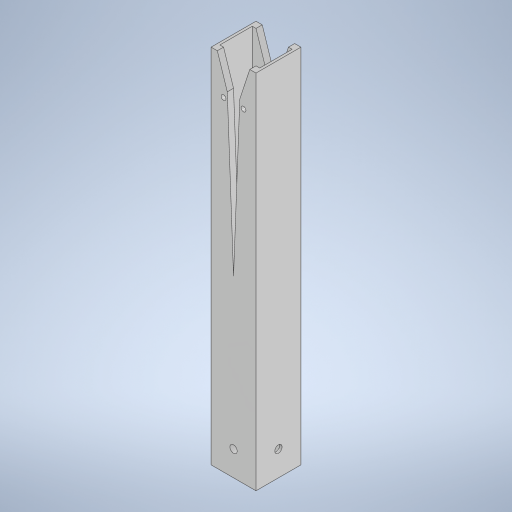
# Autodesk Inventor part: square_bar
Saved by Autodesk Inventor 2024 (Build 280153000, 153)
## iProperties
Created: 2025-01-22
Part Number: square_bar
Material: アルミニウム 6061
Document SubType Name: Modeling
Designer: 1412z
Density: 2.7 g/cm^3
Appearance: アルミニウム - つや出し
Author: 1412z
Autodesk Inventor part; units mm, degrees
ref_plane "YZ Plane" through (0, 0, 0) normal (1, 0, 0) x (0, 1, 0)
ref_plane "XZ Plane" through (0, 0, 0) normal (0, 1, 0) x (-1, 0, 0)
ref_plane "XY Plane" through (0, 0, 0) normal (0, 0, 1) x (1, 0, 0)
sketch "スケッチ1" plane through (0, 0, 0) normal (0, 1, 0) x (-1, 0, 0)
  line L0 (9, 9) -> (-9, 9)
  line L1 (-9, 9) -> (-9, -9)
  line L2 (-9, -9) -> (9, -9)
  line L3 (9, -9) -> (9, 9)
  line L4 (9, 9) -> (-9, -9) construction
  line L5 (-9, 9) -> (9, -9) construction
  point P0 (0, 0)
  dimension "d0" = 18
  dimension "d1" = 18
  constraints: 12 end point, 2 midpoint, 2 parallel, 1 horizontal, 1 perpendicular
  measures "d0" distance of L2.end L1.end
  measures "d1" distance of L1.end L0.end
extrude "押し出し1" add sketch "スケッチ1" against normal blind 150
sketch "スケッチ2" plane through (0, 0, 0) normal (0, 1, 0) x (1, 0, 0)
  line L0 (-8, -6.5) -> (8, -6.5)
  line L1 (8, -6.5) -> (8, 6.5)
  line L2 (8, 6.5) -> (-8, 6.5)
  line L3 (-8, 6.5) -> (-8, -6.5)
  line L4 (-8, -6.5) -> (8, 6.5) construction
  line L5 (8, -6.5) -> (-8, 6.5) construction
  point P0 (0, 0)
  dimension "d4" = 16
  dimension "d5" = 13
  constraints: 12 end point, 2 midpoint, 2 parallel, 1 horizontal, 1 perpendicular
  measures "d4" distance of L2.end L1.end
  measures "d5" distance of L1.end L0.end
extrude "押し出し2" cut sketch "スケッチ2" against normal blind 150
sketch "スケッチ4" plane through (-9, -150, 9) normal (0, 0, 1) x (1, 0, 0)
  circle A0 centre (5, 135) radius 1
  circle A1 centre (13, 135) radius 1
  point P0 (9, 150)
  dimension "d11" = 2
  dimension "d12" = 2
  constraints: 2 centre point
  measures "d11" diameter of A0
  measures "d12" diameter of A1
extrude "押し出し4" cut sketch "スケッチ4" against normal blind 150
sketch "スケッチ5" plane through (-9, -150, 9) normal (0, 0, 1) x (1, 0, 0)
  circle A0 centre (9, 15) radius 1.5
  point P0 (9, 150)
  dimension "d15" = 3
  constraints: 1 centre point
  measures "d15" diameter of A0
extrude "押し出し5" cut sketch "スケッチ5" against normal blind 150
sketch "スケッチ6" plane through (-9, 0, -9) normal (-1, 0, 0) x (0, 0, 1)
  circle A0 centre (9, -135) radius 1.5
  point P0 (9, 0)
  dimension "d18" = 3
  constraints: 1 centre point
  measures "d18" diameter of A0
extrude "押し出し6" cut sketch "スケッチ6" against normal blind 150
thread "ねじ1" size "M3x0.5" class "6H" standard "ANSI Metric M Profile" full length
thread "ねじ2" size "M3x0.5" class "6H" standard "ANSI Metric M Profile" full length
sketch "スケッチ7" plane through (-9, 0, 9) normal (0, 0, 1) x (1, 0, 0)
  line L0 (9, 0) -> (9, -75)
  line L1 (9, 0) -> (6, 0)
  line L2 (0, 0) -> (18, 0) projected
  line L3 (6, 0) -> (9, -75)
  line L4 (9, 0) -> (12, 0)
  line L5 (12, 0) -> (9, -75)
  point P0 (12, 0)
  dimension "d25" = 75
  dimension "d26" = 3
  dimension "d27" = 3
  constraints: 10 end point, 2 point on line, 1 vertical
  measures "d25" distance of L0.start L0.end
  measures "d26" distance of L0.start L1.end
  measures "d27" distance of L0.start L4.end
extrude "押し出し7" cut sketch "スケッチ7" against normal blind 30
sketch "スケッチ8" plane through (-9, -150, 9) normal (0, 0, 1) x (1, 0, 0)
  line L0 (9, 150) -> (15.5, 150)
  line L1 (18, 150) -> (12, 150) projected
  line L2 (9, 150) -> (9, 130)
  line L3 (9, 130) -> (15.5, 150)
  line L4 (9, 150) -> (2.5, 150)
  line L5 (2.5, 150) -> (9, 130)
  dimension "d30" = 6.5
  dimension "d31" = 20
  dimension "d32" = 6.5
  constraints: 10 end point, 1 perpendicular, 1 point on line, 1 vertical
  measures "d30" distance of L0.start L0.end
  measures "d31" distance of L0.start L2.end
  measures "d32" distance of L0.start L4.end
extrude "押し出し8" cut sketch "スケッチ8" against normal blind 30
sketch "スケッチ9" plane through (9, -150, -9) normal (0, 0, -1) x (-1, 0, 0)
  line L0 (9, 150) -> (9, 20)
  line L1 (11.5088, 137.7193) -> (9, 75) projected
  line L2 (11.5088, 137.7193) -> (11.5088, 20)
  line L3 (11.5088, 20) -> (9, 20)
  line L4 (2.5, 150) -> (6.4912, 137.7193) projected
  line L5 (6.4912, 137.7193) -> (6.4912, 20)
  line L6 (6.4912, 20) -> (9, 20)
  line L7 (6.4912, 137.7193) -> (11.5088, 137.7193)
  dimension "d35" = 130
  constraints: 12 end point, 3 perpendicular, 2 vertical, 1 parallel, 1 point on line
  measures "d35" distance of L0.start L0.end
extrude "押し出し9" cut sketch "スケッチ9" against normal blind 10
sketch "スケッチ10" plane through (0, -150, 0) normal (0, -1, 0) x (1, 0, 0)
  line L0 (-9, -9) -> (-9, 9) projected
  line L1 (9, 9) -> (-9, 9)
  line L2 (-9, 9) -> (-9, -9)
  line L3 (-9, -9) -> (9, -9)
  line L4 (9, -9) -> (9, 9)
  line L5 (9, 9) -> (-9, -9) construction
  line L6 (-9, 9) -> (9, -9) construction
  point P0 (0, 0)
  constraints: 12 end point, 2 midpoint, 2 parallel, 1 horizontal, 1 perpendicular
extrude "押し出し10" cut sketch "スケッチ10" against normal blind 5
